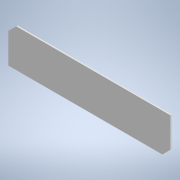
# Autodesk Inventor part: filter2
Saved by Autodesk Inventor 2022 (Build 260153000, 153)
## iProperties
Created: 2024-07-15
Part Number: filter2
Material: Типовые
Document SubType Name: Modeling
Designer: Капустяник Андрей
Density: 1 g/cm^3
Appearance: По умолчанию
Author: Капустяник Андрей
Autodesk Inventor part; units mm, degrees
ref_plane "YZ Plane" through (0, 0, 0) normal (1, 0, 0) x (0, 1, 0)
ref_plane "XZ Plane" through (0, 0, 0) normal (0, 1, 0) x (-1, 0, 0)
ref_plane "XY Plane" through (0, 0, 0) normal (0, 0, 1) x (1, 0, 0)
sketch "Эскиз1" plane through (0, 0, 0) normal (0, 0, 1) x (1, 0, 0)
  line L0 (-58.5756, 7.5) -> (-58.5756, 0.6288) projected
  line L1 (-53.5756, 12.5) -> (-58.5756, 7.5) projected
  line L2 (-46.7044, 12.5) -> (-53.5756, 12.5) projected
  line L3 (-46.7044, 12.5) -> (-58.5756, 0.6288) projected
  line L4 (-3.4075, -12.5) -> (3.4636, -12.5) projected
  line L5 (-3.4075, -12.5) -> (21.5925, 12.5) projected
  line L6 (28.4636, 12.5) -> (21.5925, 12.5) projected
  line L7 (28.4636, 12.5) -> (3.4636, -12.5) projected
  line L8 (-40.9915, -12.5) -> (-34.1204, -12.5) projected
  line L9 (-40.9915, -12.5) -> (-15.9915, 12.5) projected
  line L10 (-9.1204, 12.5) -> (-15.9915, 12.5) projected
  line L11 (-9.1204, 12.5) -> (-34.1204, -12.5) projected
  line L12 (9.1205, -12.5) -> (34.1205, 12.5) projected
  line L13 (40.9916, 12.5) -> (34.1205, 12.5) projected
  line L14 (40.9916, 12.5) -> (15.9916, -12.5) projected
  line L15 (9.1205, -12.5) -> (15.9916, -12.5) projected
  line L16 (-58.5756, -5.0281) -> (-41.0475, 12.5) projected
  line L17 (-34.1764, 12.5) -> (-41.0475, 12.5) projected
  line L18 (-34.1764, 12.5) -> (-58.5756, -11.8992) projected
  line L19 (-58.5756, -5.0281) -> (-58.5756, -11.8992) projected
  line L20 (-53.5195, -12.5) -> (-28.5195, 12.5) projected
  line L21 (-21.6484, 12.5) -> (-28.5195, 12.5) projected
  line L22 (-21.6484, 12.5) -> (-46.6484, -12.5) projected
  line L23 (-53.5195, -12.5) -> (-46.6484, -12.5) projected
  line L24 (-15.9355, -12.5) -> (-9.0644, -12.5) projected
  line L25 (-15.9355, -12.5) -> (9.0645, 12.5) projected
  line L26 (15.9356, 12.5) -> (9.0645, 12.5) projected
  line L27 (15.9356, 12.5) -> (-9.0644, -12.5) projected
  line L28 (-28.4635, -12.5) -> (-3.4635, 12.5) projected
  line L29 (3.4076, 12.5) -> (-3.4635, 12.5) projected
  line L30 (3.4076, 12.5) -> (-21.5924, -12.5) projected
  line L31 (-28.4635, -12.5) -> (-21.5924, -12.5) projected
  line L32 (58.5756, -7.5) -> (58.5756, -0.6289) projected
  line L33 (53.5756, -12.5) -> (58.5756, -7.5) projected
  line L34 (46.7045, -12.5) -> (53.5756, -12.5) projected
  line L35 (46.7045, -12.5) -> (58.5756, -0.6289) projected
  line L36 (21.6485, -12.5) -> (46.6485, 12.5) projected
  line L37 (53.5196, 12.5) -> (46.6485, 12.5) projected
  line L38 (53.5196, 12.5) -> (28.5196, -12.5) projected
  line L39 (21.6485, -12.5) -> (28.5196, -12.5) projected
  line L40 (-60.5756, -14.5) -> (-60.5756, 8.3284) projected
  line L41 (54.404, -14.5) -> (-60.5756, -14.5) projected
  line L42 (60.5756, -8.3284) -> (54.404, -14.5) projected
  line L43 (60.5756, 14.5) -> (60.5756, -8.3284) projected
  line L44 (-54.404, 14.5) -> (60.5756, 14.5) projected
  line L45 (-60.5756, 8.3284) -> (-54.404, 14.5) projected
  line L46 (58.5756, 5.028) -> (41.0476, -12.5) projected
  line L47 (34.1765, -12.5) -> (41.0476, -12.5) projected
  line L48 (34.1765, -12.5) -> (58.5756, 11.8991) projected
  line L49 (58.5756, 5.028) -> (58.5756, 11.8991) projected
  line L50 (-60.2256, -14.15) -> (-60.2256, 8.1835)
  line L51 (-60.2256, 8.1835) -> (-54.2591, 14.15)
  line L52 (-54.2591, 14.15) -> (60.2256, 14.15)
  line L53 (60.2256, 14.15) -> (60.2256, -8.1835)
  line L54 (60.2256, -8.1835) -> (54.2591, -14.15)
  line L55 (54.2591, -14.15) -> (-60.2256, -14.15)
  point P0 (0, 0)
  dimension "d0" = 0.35
  constraints: 12 end point, 5 other
  measures "d0" distance between parallel lines of L41 L55
extrude "Выдавливание1" add sketch "Эскиз1" along normal blind 1 contours L1 L2 L3 L0 | L5 L6 L7 L4 | L9 L10 L11 L8 | L12 L13 L14 L15 | L16 L17 L18 L19 | L20 L21 L22 L23 | L25 L26 L27 L24 | L28 L29 L30 L31 | L33 L34 L35 L32 | L36 L37 L38 L39 | L46 L47 L48 L49 | L50 L51 L52 L53 L54 L55
